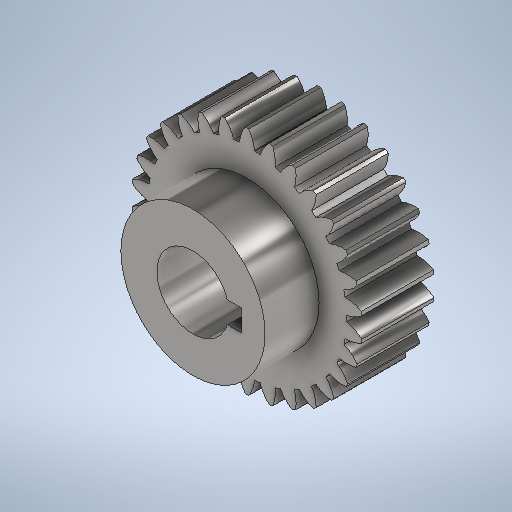
# Autodesk Inventor part: cad@70
Saved by Autodesk Inventor 2025.2 (Build 292293000, 293)
## iProperties
Created: 2025-04-22
Part Number: cad@70
Material: Generic
Document SubType Name: Modeling
Designer: spars
Density: 1 g/cm^3
Appearance: Steel - Polished
Author: spars
Autodesk Inventor part; units mm, degrees
ref_plane "YZ Plane" through (0, 0, 0) normal (1, 0, 0) x (0, 1, 0)
ref_plane "XZ Plane" through (0, 0, 0) normal (0, 1, 0) x (-1, 0, 0)
ref_plane "XY Plane" through (0, 0, 0) normal (0, 0, 1) x (1, 0, 0)
sketch "Sketch1" plane through (0, 0, 0) normal (0, 0, 1) x (1, 0, 0)
  circle A0 centre (0, 0) radius 32
  circle A1 centre (0, 0) radius 30
  circle A2 centre (0, 0) radius 27.6667
  line L0 (-27.6667, 0) -> (0, 0) construction
  line L1 (0, 0) -> (0, 27.6667) construction
  arc A3 (-0.5, 31.9961) -> (-2.1, 27.5869) centre (6.8624, 26.8296) ccw
  arc A4 (2.1, 27.5869) -> (0.5, 31.9961) centre (-6.8624, 26.8296) ccw
  point P0 (1.57, 29.9589)
  point P1 (-1.57, 29.9589)
  point P2 (2.1, 27.5869)
  point P3 (0.5, 31.9961)
  dimension "d0" = 64
  dimension "d1" = 60
  dimension "d2" = 55.3333
  dimension "d3" = 3.14
  dimension "d4" = 1
  dimension "d5" = 4.2
  constraints: 10 point on circle, 4 centre point, 4 end point, 3 coincident, 3 symmetric about line, 1 horizontal, 1 horizontal alignment, 1 perpendicular, 4 other
  measures "d1" diameter of A1
  measures "d2" diameter of A2
  measures "d3" distance of A1.end A1.start
  measures "d4" distance of A4.end A3.start
  measures "d5" distance of A4.start A3.end
extrude "Extrusion1" add sketch "Sketch1" along normal blind 20 contours A2
extrude "Extrusion2" add sketch "Sketch1" along normal blind 20 contours A4 A1 A3 A0 | A4 A2 A3 A1 picked at (-0.1745, 30.8974) picked at (-0.1745, 28.437)
fillet "Fillet1" radius 0.1 2 edges at (2.1, 27.5869, 10) (-2.1, 27.5869, 10)
pattern_circular "Circular Pattern1" count 30 over 360 about axis through (0, 0, 0) along (0, 0, 1) of "Extrusion2"
sketch "Sketch2" plane through (0, 0, 20) normal (0, 0, 1) x (1, 0, 0)
  circle A0 centre (0, 0) radius 20
  circle A1 centre (0, 0) radius 10
  dimension "d14" = 40
  dimension "d15" = 20
  constraints: 2 centre point, 2 coincident
  measures "d14" diameter of A0
  measures "d15" diameter of A1
extrude "Extrusion3" add sketch "Sketch2" along normal blind 15
sketch "Sketch3" plane through (0, 0, 20) normal (0, 0, 1) x (1, 0, 0)
  point P0 (0, 0)
sketch "Sketch4" plane through (0, 0, 20) normal (0, 0, 1) x (1, 0, 0)
  circle A0 centre (0, 0) radius 10
  dimension "d18" = 20
  constraints: 1 centre point, 1 coincident
  measures "d18" diameter of A0
extrude "Extrusion4" cut sketch "Sketch4" against normal through all
sketch "Sketch5" plane through (0, 0, 35) normal (0, 0, 1) x (1, 0, 0)
  line L0 (6.5, 3) -> (13.5, 3)
  line L1 (13.5, 3) -> (13.5, -3)
  line L2 (13.5, -3) -> (6.5, -3)
  line L3 (6.5, -3) -> (6.5, 3)
  circle A0 centre (0, 0) radius 10 projected
  line L4 (6.5, 3) -> (13.5, -3) construction
  line L5 (13.5, 3) -> (6.5, -3) construction
  point P0 (10, 0)
  dimension "d21" = 6
  dimension "d22" = 13.5
  constraints: 12 end point, 2 midpoint, 2 parallel, 1 horizontal, 1 horizontal alignment, 1 perpendicular, 1 other
  measures "d21" distance of L0.end L1.end
  measures "d22" distance from line of L1 point (0, 0)
extrude "Extrusion5" cut sketch "Sketch5" against normal through all contours L0 A0 L2 L3 | L0 L1 L2 A0 picked at (7.6667, 0)
body "Solid1"
